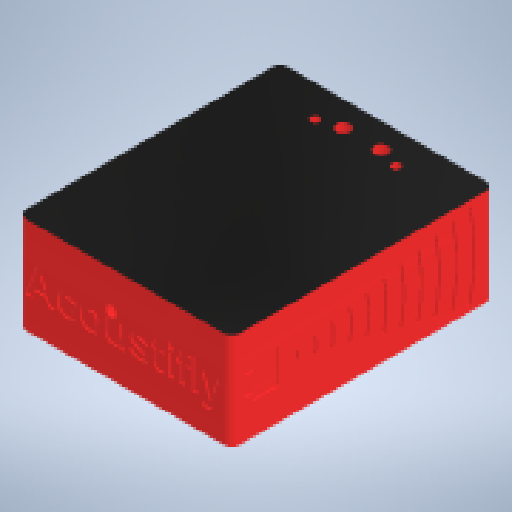
# Autodesk Inventor part: Base
Saved by Autodesk Inventor 2023.3 (Build 273359000, 359)
## iProperties
Created: 2024-05-30
Part Number: Base
Material: Generic
Document SubType Name: Modeling
Designer: Sven
Density: 1 g/cm^3
Appearance: Light Red
Author: Sven
Autodesk Inventor part; units mm, degrees
ref_plane "YZ Plane" through (0, 0, 0) normal (1, 0, 0) x (0, 1, 0)
ref_plane "XZ Plane" through (0, 0, 0) normal (0, 1, 0) x (-1, 0, 0)
ref_plane "XY Plane" through (0, 0, 0) normal (0, 0, 1) x (1, 0, 0)
sketch "Sketch1" plane through (0, 0, 0) normal (0, 1, 0) x (-1, 0, 0)
  line L0 (-25.5, 31.25) -> (25.5, 31.25)
  line L1 (25.5, 31.25) -> (25.5, -31.25)
  line L2 (25.5, -31.25) -> (-25.5, -31.25)
  line L3 (-25.5, -31.25) -> (-25.5, 31.25)
  point P0 (0, 0)
  point P1 (-25.5, 0)
  point P2 (0, -31.25)
  dimension "d0" = 62.5
  dimension "d1" = 51
  constraints: 8 end point, 2 midpoint, 2 parallel, 1 horizontal, 1 horizontal alignment, 1 perpendicular, 1 vertical alignment
  measures "d0" distance of L2.end L0.start
  measures "d1" distance of L1.end L2.end
extrude "Extrusion1" add sketch "Sketch1" along normal blind 23
fillet "Fillet1" radius 2 4 edges at (25.5, 11.5, -31.25) (25.5, 11.5, 31.25) (-25.5, 11.5, -31.25) (-25.5, 11.5, 31.25)
shell "Shell1" thickness 1.8 removed faces 1 at (-8.5, 0, -9.75)
sketch "Sketch2" plane through (-23.5, 21.2, -29.45) normal (0, -1, 0) x (1, 0, 0)
  circle A0 centre (43, 3.2) radius 2
  circle A1 centre (43, 52.2) radius 2
  circle A2 centre (4, 52.2) radius 2
  circle A3 centre (4, 3.2) radius 2
  line L0 (47, -1.8) -> (0, -1.8) projected
  line L1 (0, 60.7) -> (47, 60.7) projected
  line L2 (43, 52.2) -> (4, 52.2)
  line L3 (4, 52.2) -> (4, 3.2)
  line L4 (4, 3.2) -> (43, 3.2)
  line L5 (43, 3.2) -> (43, 52.2)
  line L6 (47, 0) -> (0, 0) projected
  line L7 (0, 58.9) -> (47, 58.9) projected
  line L8 (39, 58.9) -> (39, 52.2)
  line L9 (43, 48.2) -> (47.2, 48.2)
  line L10 (47.2, 58.7) -> (47.2, 0.2) projected
  arc A4 (39, 52.2) -> (43, 48.2) centre (43, 52.2) ccw
  line L11 (8, 58.9) -> (8, 52.2)
  line L12 (-0.2, 48.2) -> (4, 48.2)
  arc A5 (4, 48.2) -> (8, 52.2) centre (4, 52.2) ccw
  line L13 (-0.2, 0.2) -> (-0.2, 58.7) projected
  line L14 (-0.2, 7.2) -> (4, 7.2)
  line L15 (8, 3.2) -> (8, 0)
  arc A6 (8, 3.2) -> (4, 7.2) centre (4, 3.2) ccw
  line L16 (47.2, 7.2) -> (43, 7.2)
  line L17 (39, 0) -> (39, 3.2)
  arc A7 (43, 7.2) -> (39, 3.2) centre (43, 3.2) ccw
  arc A8 (47.2, 58.7) -> (47, 58.9) centre (47, 58.7) ccw projected
  line L18 (47.2, 58.7) -> (47.2, 0.2) projected
  arc A9 (47, 0) -> (47.2, 0.2) centre (47, 0.2) ccw projected
  line L19 (47, 0) -> (0, 0) projected
  arc A10 (-0.2, 0.2) -> (0, 0) centre (0, 0.2) ccw projected
  line L20 (-0.2, 0.2) -> (-0.2, 58.7) projected
  arc A11 (0, 58.9) -> (-0.2, 58.7) centre (0, 58.7) ccw projected
  line L21 (0, 58.9) -> (47, 58.9) projected
  arc A12 (0, 60.7) -> (-2, 58.7) centre (0, 58.7) ccw projected
  line L22 (-2, 0.2) -> (-2, 58.7) projected
  arc A13 (-2, 0.2) -> (0, -1.8) centre (0, 0.2) ccw projected
  line L23 (47, -1.8) -> (0, -1.8) projected
  arc A14 (47, -1.8) -> (49, 0.2) centre (47, 0.2) ccw projected
  line L24 (49, 58.7) -> (49, 0.2) projected
  arc A15 (49, 58.7) -> (47, 60.7) centre (47, 58.7) ccw projected
  line L25 (0, 60.7) -> (47, 60.7) projected
  point P0 (23.5, 29.45)
  point P1 (23.5, 3.2)
  point P2 (23.5, 0)
  point P3 (-0.2, 0.2)
  point P4 (47.2, 0.2)
  point P5 (47, 58.9)
  point P6 (0, 58.9)
  point P7 (-0.2, 58.7)
  dimension "d6" = 4
  dimension "d7" = 5
  dimension "d9" = 8.5
  dimension "d10" = 39
  dimension "d11" = 2
  dimension "d12" = 2
  dimension "d13" = 2
  dimension "d14" = 2
  constraints: 24 end point, 15 point on line, 8 centre point, 8 perpendicular, 8 point on circle, 4 concentric, 3 equal radius, 2 coincident, 2 horizontal, 2 horizontal alignment, 2 midpoint, 2 parallel, 2 vertical alignment
  measures "d6" diameter of A1
  measures "d7" distance from line of L0 A0.centre
  measures "d9" distance from line of L1 L2.start
  measures "d10" distance of L2.start L2.end
  measures "d11" radial gap between concentric circles of A4 A1
  measures "d12" radial gap between concentric circles of A2 A5
  measures "d13" radial gap between concentric circles of A3 A6
  measures "d14" radial gap between concentric circles of A7 A0
extrude "Extrusion2" add sketch "Sketch2" along normal blind 4.5 contours A0 L5 L16 L10 A9 L6 L17 L4 | A0 L4 A7 L5 | A4 L2 A1 L5 | L5 A1 L2 L8 L7 A8 L10 L9 | L15 L6 A10 L13 L14 L3 A3 L4 | L4 A3 L3 A6 | A5 L3 A2 L2 | L2 A2 L3 L12 L13 A11 L7 L11
sketch "Sketch3" plane through (23.5, 0, -31.25) normal (0, 0, -1) x (-1, 0, 0)
  line L0 (17.3204, 15.3186) -> (10.8612, 15.3213)
  arc A0 (10.8612, 15.3213) -> (9.405, 13.995) centre (10.8606, 13.8594) ccw
  line L1 (9.405, 13.995) -> (9.405, 13.0849)
  arc A1 (9.405, 13.0849) -> (10.8624, 11.7368) centre (10.8624, 13.1987) ccw
  line L2 (10.8624, 11.7368) -> (17.4454, 11.7368)
  arc A2 (17.4454, 11.7368) -> (18.7701, 13.0614) centre (17.3031, 13.2038) ccw
  line L3 (18.7701, 13.0614) -> (18.7701, 13.9715)
  arc A3 (18.7701, 13.9715) -> (17.3204, 15.3186) centre (17.3198, 13.8644) ccw
  line L4 (10.8613, 15.7213) -> (17.3206, 15.7186)
  arc A4 (19.1701, 13.9853) -> (17.3206, 15.7186) centre (17.3198, 13.8644) ccw
  line L5 (19.1701, 13.9853) -> (19.1701, 13.0432)
  arc A5 (17.4636, 11.3368) -> (19.1701, 13.0432) centre (17.3031, 13.2038) ccw
  line L6 (17.4636, 11.3368) -> (10.8624, 11.3368)
  arc A6 (9.005, 13.0703) -> (10.8624, 11.3368) centre (10.8624, 13.1987) ccw
  line L7 (9.005, 13.0703) -> (9.005, 14.0124)
  arc A7 (10.8613, 15.7213) -> (9.005, 14.0124) centre (10.8606, 13.8594) ccw
  point P0 (23.5, 0)
  dimension "d20" = 1.4542
  dimension "d21" = 1.4739
  dimension "d22" = 1.4619
  dimension "d23" = 90.024
  dimension "d24" = 9.3651
  dimension "d25" = 4.7299
  dimension "d26" = 11.7368
  dimension "d27" = 15.3161
  dimension "d28" = 2.2346
  dimension "d29" = 1.3246
  dimension "d30" = 1.3246
  dimension "d31" = 7.9077
  dimension "d32" = 7.9089
  dimension "d121" = 0.4
  constraints: 16 end point, 16 point on circle, 8 centre point, 3 tangent, 2 parallel, 2 perpendicular, 1 equal radius, 1 horizontal, 7 other
  measures "d20" radius of A3
  measures "d21" radius of A2
  measures "d22" radius of A1
  measures "d23" angle of L3 L0
  measures "d24" distance between parallel lines of L3 L1
  measures "d25" distance from line of point (23.5, 0) L3
  measures "d26" distance from line of point (23.5, 0) L2
  measures "d27" distance from line of point (23.5, 0) L0
  measures "d28" distance from line of L3.end L2
  measures "d29" distance from line of L3.start L2
  measures "d30" distance from line of L2.end L3
  measures "d31" distance from line of A1.centre L3
  measures "d32" distance from line of L0.end L3
  measures "d121" distance between parallel lines of L0 L4
extrude "Extrusion4" cut sketch "Sketch3" against normal blind 10 contours A3 L3 A2 L2 A1 L1 A0 L0
sketch "Sketch4" plane through (0, 23, 0) normal (0, 1, 0) x (1, 0, 0)
  circle A0 centre (-4.5, 25.25) radius 1.65
  circle A1 centre (4.5, 25.25) radius 1.65
  line L0 (23.5, 31.25) -> (-23.5, 31.25) projected
  line L1 (-4.5, 25.25) -> (4.5, 25.25)
  point P0 (0, 0)
  point P1 (0, 25.25)
  point P2 (0, 31.25)
  dimension "d35" = 3.3
  dimension "d36" = 9
  dimension "d37" = 6
  constraints: 2 centre point, 2 end point, 2 midpoint, 1 equal radius, 1 horizontal, 1 horizontal alignment, 1 vertical alignment
  measures "d35" diameter of A0
  measures "d36" distance of L1.end L1.start
  measures "d37" distance from line of L0 L1.start
extrude "Extrusion5" cut sketch "Sketch4" against normal blind 10
sketch "Sketch5" plane through (23.5, 0, -31.25) normal (0, 0, -1) x (-1, 0, 0)
  line L0 (28.4701, 14.4) -> (35.4701, 14.4)
  line L1 (35.4701, 14.4) -> (35.4701, 10.6)
  line L2 (35.4701, 10.6) -> (28.4701, 10.6)
  line L3 (28.4701, 10.6) -> (28.4701, 14.4)
  line L4 (0, 16.7) -> (8, 16.7) projected
  line L5 (39, 16.7) -> (47, 16.7) projected
  line L6 (18.7701, 13.9715) -> (18.7701, 13.0614) projected
  point P0 (23.5, 0)
  point P1 (18.7701, 13.5164)
  dimension "d40" = 2.3
  dimension "d41" = 6.1
  dimension "d42" = 7
  dimension "d43" = 9.7
  constraints: 8 end point, 2 parallel, 1 horizontal, 1 midpoint, 1 perpendicular
  measures "d40" distance between parallel lines of L5 L0
  measures "d41" distance between parallel lines of L2 L5
  measures "d42" distance of L1.end L2.end
  measures "d43" distance from line of point (18.77, 13.516) L3
extrude "Extrusion6" cut sketch "Sketch5" against normal blind 10
sketch "Sketch6" plane through (23.5, 0, -31.25) normal (0, 0, -1) x (-1, 0, 0)
  circle A0 centre (22.3701, 14.3165) radius 0.75
  line L0 (10.8612, 15.3213) -> (17.3204, 15.3186) projected
  line L1 (18.7701, 13.9715) -> (18.7701, 13.0614) projected
  point P0 (23.5, 0)
  point P1 (18.7701, 13.5164)
  dimension "d46" = 1.5
  dimension "d47" = 1
  dimension "d48" = 3.6
  constraints: 1 centre point, 1 midpoint
  measures "d46" diameter of A0
  measures "d47" distance from line of A0.centre L0
  measures "d48" horizontal distance of point (18.77, 13.516) A0.centre
extrude "Extrusion7" cut sketch "Sketch6" against normal blind 10
sketch "Sketch7" plane through (-23.5, 0, 31.25) normal (0, 0, 1) x (1, 0, 0)
  circle A0 centre (20.2, 14.07) radius 1.25
  line L0 (1, 15.12) -> (7.002, 15.12) projected
  line L1 (0, 16.7) -> (-0.2, 16.7) projected
  line L2 (8, 16.7) -> (0, 16.7) projected
  line L3 (8, 16.7) -> (4, 16.7) projected
  line L4 (4, 16.7) -> (-0.2, 16.7) projected
  line L5 (6, 16.7) -> (2, 16.7) projected
  point P0 (23.5, 0)
  dimension "d51" = 19.2
  dimension "d52" = 2.5
  dimension "d53" = 1.05
  constraints: 1 centre point
  measures "d51" horizontal distance of A0.centre L0.start
  measures "d52" diameter of A0
  measures "d53" distance from line of A0.centre L0
extrude "Extrusion8" cut sketch "Sketch7" against normal blind 10
sketch "Sketch8" plane through (0, 0, 0) normal (0, -1, 0) x (1, 0, 0)
  line L0 (23.5, -29.45) -> (-23.5, -29.45) projected
  line L1 (19.2, -29.45) -> (23.7, -24.95)
  line L2 (23.7, 29.25) -> (23.7, -29.25) projected
  arc A0 (23.7, 29.25) -> (23.5, 29.45) centre (23.5, 29.25) ccw projected
  line L3 (23.7, 29.25) -> (23.7, -29.25) projected
  arc A1 (23.5, -29.45) -> (23.7, -29.25) centre (23.5, -29.25) ccw projected
  line L4 (23.5, -29.45) -> (-23.5, -29.45) projected
  arc A2 (-23.7, -29.25) -> (-23.5, -29.45) centre (-23.5, -29.25) ccw projected
  line L5 (-23.7, -29.25) -> (-23.7, 29.25) projected
  arc A3 (-23.5, 29.45) -> (-23.7, 29.25) centre (-23.5, 29.25) ccw projected
  line L6 (-23.5, 29.45) -> (23.5, 29.45) projected
  arc A4 (-23.5, 31.25) -> (-25.5, 29.25) centre (-23.5, 29.25) ccw projected
  line L7 (-25.5, -29.25) -> (-25.5, 29.25) projected
  arc A5 (-25.5, -29.25) -> (-23.5, -31.25) centre (-23.5, -29.25) ccw projected
  line L8 (23.5, -31.25) -> (-23.5, -31.25) projected
  arc A6 (23.5, -31.25) -> (25.5, -29.25) centre (23.5, -29.25) ccw projected
  line L9 (25.5, 29.25) -> (25.5, -29.25) projected
  arc A7 (25.5, 29.25) -> (23.5, 31.25) centre (23.5, 29.25) ccw projected
  line L10 (-23.5, 31.25) -> (23.5, 31.25) projected
  line L11 (23.7, 24.95) -> (19.2, 29.45)
  line L12 (-23.7, 24.95) -> (-19.2, 29.45)
  line L13 (-19.2, -29.45) -> (-23.7, -24.95)
  point P0 (0, 0)
  point P1 (23.7, -29.25)
  point P2 (-19.2, -29.45)
  dimension "d56" = 4.5
  dimension "d57" = 4.5
  dimension "d58" = 4.5
  dimension "d59" = 4.5
  dimension "d60" = 4.5
  dimension "d61" = 4.5
  dimension "d62" = 4.5
  dimension "d63" = 4.5
  constraints: 8 end point, 8 point on line
  measures "d56" distance from line of L2 L1.start
  measures "d57" distance from line of L0 L1.end
  measures "d58" distance from line of L6 L11.start
  measures "d59" distance from line of L2 L11.end
  measures "d60" distance from line of L5 L12.end
  measures "d61" distance from line of L6 L12.start
  measures "d62" distance from line of L5 L13.start
  measures "d63" distance from line of L0 L13.end
extrude "Extrusion9" add sketch "Sketch8" against normal blind 4 contours L0 L1 L2 A1 | L0 A2 L5 L13 | L11 L6 A0 L2 | L5 A3 L6 L12
sketch "Sketch9" plane through (0, 0, 0) normal (0, -1, 0) x (1, 0, 0)
  line L0 (-23.7, -29.25) -> (-23.7, -22.25) projected
  arc A0 (-23.7, -29.25) -> (-23.5, -29.45) centre (-23.5, -29.25) ccw projected
  line L1 (-15.5, -29.45) -> (-23.5, -29.45) projected
  line L2 (-15.5, -29.45) -> (-15.5, -26.25) projected
  arc A1 (-15.5, -26.25) -> (-19.5, -22.25) centre (-19.5, -26.25) ccw projected
  line L3 (-19.5, -22.25) -> (-23.7, -22.25) projected
  circle A2 centre (-19.5, -26.25) radius 2 projected
  line L4 (23.7, 24.95) -> (23.7, -24.95) projected
  line L5 (23.7, -24.95) -> (19.2, -29.45) projected
  line L6 (19.2, -29.45) -> (-19.2, -29.45) projected
  line L7 (-19.2, -29.45) -> (-23.7, -24.95) projected
  line L8 (-23.7, -24.95) -> (-23.7, 24.95) projected
  line L9 (-23.7, 24.95) -> (-19.2, 29.45) projected
  line L10 (-19.2, 29.45) -> (19.2, 29.45) projected
  line L11 (19.2, 29.45) -> (23.7, 24.95) projected
  arc A3 (-23.5, 31.25) -> (-25.5, 29.25) centre (-23.5, 29.25) ccw projected
  line L12 (-25.5, -29.25) -> (-25.5, 29.25) projected
  arc A4 (-25.5, -29.25) -> (-23.5, -31.25) centre (-23.5, -29.25) ccw projected
  line L13 (23.5, -31.25) -> (-23.5, -31.25) projected
  arc A5 (23.5, -31.25) -> (25.5, -29.25) centre (23.5, -29.25) ccw projected
  line L14 (25.5, 29.25) -> (25.5, -29.25) projected
  arc A6 (25.5, 29.25) -> (23.5, 31.25) centre (23.5, 29.25) ccw projected
  line L15 (-23.5, 31.25) -> (23.5, 31.25) projected
  line L16 (23.5, -29.45) -> (15.5, -29.45) projected
  arc A7 (23.5, -29.45) -> (23.7, -29.25) centre (23.5, -29.25) ccw projected
  line L17 (23.7, -22.25) -> (23.7, -29.25) projected
  line L18 (23.7, -22.25) -> (19.5, -22.25) projected
  arc A8 (19.5, -22.25) -> (15.5, -26.25) centre (19.5, -26.25) ccw projected
  line L19 (15.5, -26.25) -> (15.5, -29.45) projected
  circle A9 centre (19.5, -26.25) radius 2 projected
  line L20 (23.7, 29.25) -> (23.7, 18.75) projected
  arc A10 (23.7, 29.25) -> (23.5, 29.45) centre (23.5, 29.25) ccw projected
  line L21 (15.5, 29.45) -> (23.5, 29.45) projected
  line L22 (15.5, 29.45) -> (15.5, 22.75) projected
  arc A11 (15.5, 22.75) -> (19.5, 18.75) centre (19.5, 22.75) ccw projected
  line L23 (19.5, 18.75) -> (23.7, 18.75) projected
  circle A12 centre (19.5, 22.75) radius 2 projected
  line L24 (-23.5, 29.45) -> (-15.5, 29.45) projected
  arc A13 (-23.5, 29.45) -> (-23.7, 29.25) centre (-23.5, 29.25) ccw projected
  line L25 (-23.7, 18.75) -> (-23.7, 29.25) projected
  line L26 (-23.7, 18.75) -> (-19.5, 18.75) projected
  arc A14 (-19.5, 18.75) -> (-15.5, 22.75) centre (-19.5, 22.75) ccw projected
  line L27 (-15.5, 22.75) -> (-15.5, 29.45) projected
  circle A15 centre (-19.5, 22.75) radius 2 projected
  point P0 (0, 0)
  point P1 (23.7, -24.95)
  point P2 (19.2, -29.45)
  point P3 (19.2, 29.45)
  point P4 (-19.2, 29.45)
extrude "Extrusion10" cut sketch "Sketch9" against normal blind 2 contours L0 L7 L1 A0 | L25 A13 L24 L9 | L5 L17 A7 L16 | L21 A10 L20 L11
sketch "Sketch12" plane through (0, 23, 0) normal (0, 1, 0) x (1, 0, 0)
  circle A0 centre (-9.6, 23.75) radius 1.1 projected
  circle A1 centre (9.6, 23.75) radius 1.1 projected
  point P0 (0, 0)
extrude "Extrusion13" cut sketch "Sketch12" against normal through all
sketch "Sketch10" plane through (-23.5, 0, 31.25) normal (0, 0, 1) x (1, 0, 0)
  line L0 (-0.133, 14.659) -> (47.133, 14.659) construction
  line L1 (47.133, 14.659) -> (47.133, 5.4822) construction
  line L2 (47.133, 5.4822) -> (-0.133, 5.4822) construction
  line L3 (-0.133, 5.4822) -> (-0.133, 14.659) construction
  line L4 (0, 23) -> (47, 23) projected
  line L5 (6.8883, 7.5417) -> (5.3518, 7.5417)
  line L6 (5.3518, 7.5417) -> (4.7435, 9.1316)
  line L7 (4.7435, 9.1316) -> (1.9478, 9.1316)
  line L8 (1.9478, 9.1316) -> (1.3662, 7.5417)
  line L9 (1.3662, 7.5417) -> (-0.133, 7.5417)
  line L10 (-0.133, 7.5417) -> (2.588, 14.5417)
  line L11 (2.588, 14.5417) -> (4.0926, 14.5417)
  line L12 (4.0926, 14.5417) -> (6.8883, 7.5417)
  line L13 (4.29, 10.3161) -> (3.3243, 12.909)
  line L14 (3.3243, 12.909) -> (2.3746, 10.3161)
  line L15 (2.3746, 10.3161) -> (4.29, 10.3161)
  line L16 (12.0476, 11.1164) -> (10.7245, 10.8763)
  spline S0 degree 2 poles (10.7245, 10.8763) (10.6604, 11.2711) (10.1856, 11.6712) (9.8068, 11.6712) knots 0 0 0 1 2 2 2
  spline S1 degree 2 poles (9.8068, 11.6712) (9.3106, 11.6712) (8.713, 10.9776) (8.713, 10.1667) knots 0 0 0 1 2 2 2
  spline S2 degree 2 poles (8.713, 10.1667) (8.713, 9.265) (9.3213, 8.5234) (9.8281, 8.5234) knots 0 0 0 1 2 2 2
  spline S3 degree 2 poles (9.8281, 8.5234) (10.2123, 8.5234) (10.6978, 8.9609) (10.7992, 9.4891) knots 0 0 0 1 2 2 2
  line L17 (10.7992, 9.4891) -> (12.117, 9.265)
  spline S4 degree 2 poles (12.117, 9.265) (11.9143, 8.358) (10.7458, 7.4296) (9.7694, 7.4296) knots 0 0 0 1 2 2 2
  spline S5 degree 2 poles (9.7694, 7.4296) (8.6597, 7.4296) (7.3365, 8.8328) (7.3365, 10.076) knots 0 0 0 1 2 2 2
  spline S6 degree 2 poles (7.3365, 10.076) (7.3365, 11.3298) (8.6597, 12.7276) (9.7908, 12.7276) knots 0 0 0 1 2 2 2
  spline S7 degree 2 poles (9.7908, 12.7276) (10.7191, 12.7276) (11.8075, 11.9327) (12.0476, 11.1164) knots 0 0 0 1 2 2 2
  spline S8 degree 2 poles (12.7572, 10.1507) (12.7572, 10.8176) (13.4188, 12.0714) (14.6246, 12.7276) (15.3716, 12.7276) knots 0 0 0 1 2 3 3 3
  spline S9 degree 2 poles (15.3716, 12.7276) (16.524, 12.7276) (17.9966, 11.2337) (17.9966, 10.092) knots 0 0 0 1 2 2 2
  spline S10 degree 2 poles (17.9966, 10.092) (17.9966, 8.9449) (16.508, 7.4296) (15.3822, 7.4296) knots 0 0 0 1 2 2 2
  spline S11 degree 2 poles (15.3822, 7.4296) (14.6833, 7.4296) (13.4188, 8.0592) (12.7572, 9.2757) (12.7572, 10.1507) knots 0 0 0 1 2 3 3 3
  spline S12 degree 2 poles (14.1338, 10.0813) (14.1338, 9.3237) (14.8487, 8.5234) (15.3769, 8.5234) knots 0 0 0 1 2 2 2
  spline S13 degree 2 poles (15.3769, 8.5234) (15.9051, 8.5234) (16.6147, 9.3237) (16.6147, 10.0866) knots 0 0 0 1 2 2 2
  spline S14 degree 2 poles (16.6147, 10.0866) (16.6147, 10.8336) (15.9051, 11.6339) (15.3769, 11.6339) knots 0 0 0 1 2 2 2
  spline S15 degree 2 poles (15.3769, 11.6339) (14.8487, 11.6339) (14.1338, 10.8336) (14.1338, 10.0813) knots 0 0 0 1 2 2 2
  line L18 (22.3822, 7.5417) -> (22.3822, 8.2993)
  spline S16 degree 2 poles (22.3822, 8.2993) (22.1048, 7.8938) (21.2031, 7.4296) (20.7016, 7.4296) knots 0 0 0 1 2 2 2
  spline S17 degree 2 poles (20.7016, 7.4296) (20.1894, 7.4296) (19.3784, 7.8778) (19.0156, 8.6888) (19.0156, 9.409) knots 0 0 0 1 2 3 3 3
  line L19 (19.0156, 9.409) -> (19.0156, 12.6156)
  line L20 (19.0156, 12.6156) -> (20.3601, 12.6156)
  line L21 (20.3601, 12.6156) -> (20.3601, 10.284)
  spline S18 degree 2 poles (20.3601, 10.284) (20.3601, 9.217) (20.5095, 8.7368) (20.899, 8.454) (21.1978, 8.454) knots 0 0 0 1 2 3 3 3
  spline S19 degree 2 poles (21.1978, 8.454) (21.5446, 8.454) (22.0835, 8.8328) (22.2862, 9.3877) (22.2862, 10.4761) knots 0 0 0 1 2 3 3 3
  line L22 (22.2862, 10.4761) -> (22.2862, 12.6156)
  line L23 (22.2862, 12.6156) -> (23.6307, 12.6156)
  line L24 (23.6307, 12.6156) -> (23.6307, 7.5417)
  line L25 (23.6307, 7.5417) -> (22.3822, 7.5417)
  line L26 (24.5484, 8.9929) -> (25.8929, 9.1956)
  spline S20 degree 2 poles (25.8929, 9.1956) (25.9783, 8.8061) (26.5065, 8.4007) (26.976, 8.4007) knots 0 0 0 1 2 2 2
  spline S21 degree 2 poles (26.976, 8.4007) (27.4989, 8.4007) (27.7603, 8.5927) knots 0 0 0 1 1 1
  spline S22 degree 2 poles (27.7603, 8.5927) (27.9364, 8.7261) (27.9364, 8.9502) knots 0 0 0 1 1 1
  spline S23 degree 2 poles (27.9364, 8.9502) (27.9364, 9.0996) (27.8403, 9.201) knots 0 0 0 1 1 1
  spline S24 degree 2 poles (27.8403, 9.201) (27.7389, 9.297) (27.3921, 9.377) knots 0 0 0 1 1 1
  spline S25 degree 2 poles (27.3921, 9.377) (25.7702, 9.7345) (25.338, 10.0333) knots 0 0 0 1 1 1
  spline S26 degree 2 poles (25.338, 10.0333) (24.7351, 10.4441) (24.7351, 11.1697) knots 0 0 0 1 1 1
  spline S27 degree 2 poles (24.7351, 11.1697) (24.7351, 11.8313) (25.7755, 12.7276) (26.8693, 12.7276) knots 0 0 0 1 2 2 2
  spline S28 degree 2 poles (26.8693, 12.7276) (27.9097, 12.7276) (28.9181, 12.05) (29.1101, 11.3831) knots 0 0 0 1 2 2 2
  line L27 (29.1101, 11.3831) -> (27.8457, 11.1484)
  spline S29 degree 2 poles (27.8457, 11.1484) (27.7656, 11.4472) (27.3121, 11.7619) (26.8906, 11.7619) knots 0 0 0 1 2 2 2
  spline S30 degree 2 poles (26.8906, 11.7619) (26.3624, 11.7619) (26.1383, 11.6125) knots 0 0 0 1 1 1
  spline S31 degree 2 poles (26.1383, 11.6125) (25.9836, 11.5112) (25.9836, 11.3404) knots 0 0 0 1 1 1
  spline S32 degree 2 poles (25.9836, 11.3404) (25.9836, 11.2017) (26.117, 11.1004) knots 0 0 0 1 1 1
  spline S33 degree 2 poles (26.117, 11.1004) (26.2984, 10.967) (28.4379, 10.4815) (28.8594, 10.124) knots 0 0 0 1 2 2 2
  spline S34 degree 2 poles (28.8594, 10.124) (29.2809, 9.7665) (29.2809, 9.1263) knots 0 0 0 1 1 1
  spline S35 degree 2 poles (29.2809, 9.1263) (29.2809, 8.4327) (28.1178, 7.4296) (26.976, 7.4296) knots 0 0 0 1 2 2 2
  spline S36 degree 2 poles (26.976, 7.4296) (25.9409, 7.4296) (24.7351, 8.2726) (24.5484, 8.9929) knots 0 0 0 1 2 2 2
  line L28 (32.7809, 12.6156) -> (32.7809, 11.5485)
  line L29 (32.7809, 11.5485) -> (31.8632, 11.5485)
  line L30 (31.8632, 11.5485) -> (31.8632, 9.5051)
  spline S37 degree 2 poles (31.8632, 9.5051) (31.8632, 8.8862) (31.9165, 8.6781) (32.1033, 8.5447) (32.2367, 8.5447) knots 0 0 0 1 2 3 3 3
  spline S38 degree 2 poles (32.2367, 8.5447) (32.4234, 8.5447) (32.7809, 8.6728) knots 0 0 0 1 1 1
  line L31 (32.7809, 8.6728) -> (32.8929, 7.6324)
  spline S39 degree 2 poles (32.8929, 7.6324) (32.4234, 7.4296) (31.8312, 7.4296) knots 0 0 0 1 1 1
  spline S40 degree 2 poles (31.8312, 7.4296) (31.4684, 7.4296) (30.8868, 7.675) (30.6147, 8.0592) (30.5614, 8.39) knots 0 0 0 1 2 3 3 3
  spline S41 degree 2 poles (30.5614, 8.39) (30.5187, 8.6247) (30.5187, 9.3343) knots 0 0 0 1 1 1
  line L32 (30.5187, 9.3343) -> (30.5187, 11.5485)
  line L33 (30.5187, 11.5485) -> (29.9051, 11.5485)
  line L34 (29.9051, 11.5485) -> (29.9051, 12.6156)
  line L35 (29.9051, 12.6156) -> (30.5187, 12.6156)
  line L36 (30.5187, 12.6156) -> (30.5187, 13.624)
  line L37 (30.5187, 13.624) -> (31.8632, 14.4136)
  line L38 (31.8632, 14.4136) -> (31.8632, 12.6156)
  line L39 (31.8632, 12.6156) -> (32.7809, 12.6156)
  line L40 (33.7146, 7.5417) -> (33.7146, 12.6156)
  line L41 (33.7146, 12.6156) -> (35.0591, 12.6156)
  line L42 (35.0591, 12.6156) -> (35.0591, 7.5417)
  line L43 (35.0591, 7.5417) -> (33.7146, 7.5417)
  line L44 (33.7146, 13.2985) -> (33.7146, 14.5417)
  line L45 (33.7146, 14.5417) -> (35.0591, 14.5417)
  line L46 (35.0591, 14.5417) -> (35.0591, 13.2985)
  line L47 (35.0591, 13.2985) -> (33.7146, 13.2985)
  line L48 (35.838, 12.6156) -> (36.585, 12.6156)
  line L49 (36.585, 12.6156) -> (36.585, 12.9944)
  spline S42 degree 2 poles (36.585, 12.9944) (36.585, 13.6347) (36.8571, 14.2642) (37.588, 14.659) (38.1482, 14.659) knots 0 0 0 1 2 3 3 3
  spline S43 degree 2 poles (38.1482, 14.659) (38.7245, 14.659) (39.274, 14.4883) knots 0 0 0 1 1 1
  line L50 (39.274, 14.4883) -> (39.0926, 13.56)
  spline S44 degree 2 poles (39.0926, 13.56) (38.7725, 13.6347) (38.4737, 13.6347) knots 0 0 0 1 1 1
  spline S45 degree 2 poles (38.4737, 13.6347) (38.1803, 13.6347) (37.9295, 13.3625) (37.9295, 12.9731) knots 0 0 0 1 2 2 2
  line L51 (37.9295, 12.9731) -> (37.9295, 12.6156)
  line L52 (37.9295, 12.6156) -> (38.9325, 12.6156)
  line L53 (38.9325, 12.6156) -> (38.9325, 11.5592)
  line L54 (38.9325, 11.5592) -> (37.9295, 11.5592)
  line L55 (37.9295, 11.5592) -> (37.9295, 7.5417)
  line L56 (37.9295, 7.5417) -> (36.585, 7.5417)
  line L57 (36.585, 7.5417) -> (36.585, 11.5592)
  line L58 (36.585, 11.5592) -> (35.838, 11.5592)
  line L59 (35.838, 11.5592) -> (35.838, 12.6156)
  line L60 (39.6848, 7.5417) -> (39.6848, 14.5417)
  line L61 (39.6848, 14.5417) -> (41.0293, 14.5417)
  line L62 (41.0293, 14.5417) -> (41.0293, 7.5417)
  line L63 (41.0293, 7.5417) -> (39.6848, 7.5417)
  line L64 (41.7656, 12.6156) -> (43.1955, 12.6156)
  line L65 (43.1955, 12.6156) -> (44.412, 9.0142)
  line L66 (44.412, 9.0142) -> (45.5911, 12.6156)
  line L67 (45.5911, 12.6156) -> (46.9783, 12.6156)
  line L68 (46.9783, 12.6156) -> (45.1963, 7.7284)
  line L69 (45.1963, 7.7284) -> (44.8708, 6.8481)
  spline S46 degree 2 poles (44.8708, 6.8481) (44.6947, 6.4052) (44.3746, 5.9357) (43.9585, 5.6423) (43.3502, 5.4822) (42.9661, 5.4822) knots 0 0 0 1 2 3 4 4 4
  spline S47 degree 2 poles (42.9661, 5.4822) (42.5819, 5.4822) (42.2085, 5.5622) knots 0 0 0 1 1 1
  line L70 (42.2085, 5.5622) -> (42.0911, 6.6133)
  spline S48 degree 2 poles (42.0911, 6.6133) (42.4059, 6.5493) (42.662, 6.5493) knots 0 0 0 1 1 1
  spline S49 degree 2 poles (42.662, 6.5493) (43.1261, 6.5493) (43.5796, 7.0988) (43.697, 7.5257) knots 0 0 0 1 2 2 2
  line L71 (43.697, 7.5257) -> (41.7656, 12.6156)
  point P0 (23.5, 0)
  point P1 (23.5, 14.659)
  point P2 (23.5, 23)
  dimension "d0" = 62.5
  dimension "d1" = 51
  dimension "d68" = 47.266
  dimension "d69" = 9.1768
  dimension "d70" = 8.341
  constraints: 2 midpoint, 1 vertical alignment, 2 other
  measures "d68" distance of L1.end L2.end
  measures "d69" distance of L2.end L0.start
  measures "d70" distance between parallel lines of L4 L0
extrude "Extrusion11" cut sketch "Sketch10" against normal blind 0.4
sketch "Sketch11" plane through (25.5, 0, 29.25) normal (1, 0, 0) x (0, 0, -1)
  line L0 (9.25, 7.75) -> (9.25, 15.25)
  line L1 (9, 15.5) -> (3.25, 15.5)
  line L2 (3, 15.25) -> (3, 7.75)
  line L3 (3.25, 7.5) -> (9, 7.5)
  arc A0 (3.25, 15.5) -> (3, 15.25) centre (3.25, 15.25) ccw
  arc A1 (9.25, 15.25) -> (9, 15.5) centre (9, 15.25) ccw
  arc A2 (9, 7.5) -> (9.25, 7.75) centre (9, 7.75) ccw
  arc A3 (3, 7.75) -> (3.25, 7.5) centre (3.25, 7.75) ccw
  line L4 (3, 14) -> (1, 14)
  line L5 (1, 14) -> (1, 13.5)
  line L6 (1, 13.5) -> (3, 13.5)
  line L7 (3, 9.5) -> (1, 9.5)
  line L8 (1, 9.5) -> (1, 9)
  line L9 (1, 9) -> (3, 9)
  circle A4 centre (9.25, 11.5) radius 4.2
  circle A5 centre (9.25, 11.5) radius 4.7
  circle A6 centre (9.25, 11.5) radius 8.4
  circle A7 centre (9.25, 11.5) radius 8.9
  circle A8 centre (9.25, 11.5) radius 12.6
  circle A9 centre (9.25, 11.5) radius 13.1
  circle A10 centre (9.25, 11.5) radius 16.8
  circle A11 centre (9.25, 11.5) radius 17.3
  circle A12 centre (9.25, 11.5) radius 21
  circle A13 centre (9.25, 11.5) radius 21.5
  circle A14 centre (9.25, 11.5) radius 25.2
  circle A15 centre (9.25, 11.5) radius 25.7
  circle A16 centre (9.25, 11.5) radius 29.4
  circle A17 centre (9.25, 11.5) radius 29.9
  circle A18 centre (9.25, 11.5) radius 33.6
  circle A19 centre (9.25, 11.5) radius 34.1
  circle A20 centre (9.25, 11.5) radius 37.8
  circle A21 centre (9.25, 11.5) radius 38.3
  circle A22 centre (9.25, 11.5) radius 42
  circle A23 centre (9.25, 11.5) radius 42.5
  circle A24 centre (9.25, 11.5) radius 46.2
  circle A25 centre (9.25, 11.5) radius 46.7
  line L10 (0, 0) -> (58.5, 0) projected
  line L11 (0, 23) -> (58.5, 23) projected
  line L12 (60.5, 0) -> (60.5, 23) projected
  line L13 (9.25, 11.5) -> (60.5, 23)
  line L14 (9.25, 11.5) -> (60.5, 0)
  point P0 (29.25, 0)
  point P1 (-7, 28.5)
  point P2 (9.25, 7.5)
  point P3 (3, 15.5)
  point P4 (9.25, 15.5)
  point P5 (9.25, 11.5)
  point P6 (1, 13.75)
  point P7 (13.3481, 10.5804)
  point P8 (13.836, 10.471)
  point P9 (13.836, 12.529)
  point P10 (13.3481, 12.4196)
  point P11 (17.4462, 9.6609)
  point P12 (17.9341, 9.5514)
  point P13 (17.9341, 13.4486)
  point P14 (17.4462, 13.3391)
  point P15 (21.5443, 8.7413)
  point P16 (22.0322, 8.6318)
  point P17 (22.0322, 14.3682)
  point P18 (21.5443, 14.2587)
  point P19 (25.6424, 7.8217)
  point P20 (26.1303, 7.7122)
  point P21 (26.1303, 15.2878)
  point P22 (25.6424, 15.1783)
  point P23 (29.7405, 6.9021)
  point P24 (30.2283, 6.7927)
  point P25 (30.2283, 16.2073)
  point P26 (29.7405, 16.0979)
  point P27 (33.8386, 5.9826)
  point P28 (34.3264, 5.8731)
  point P29 (34.3264, 17.1269)
  point P30 (33.8386, 17.0174)
  point P31 (37.9367, 5.063)
  point P32 (38.4245, 4.9535)
  point P33 (38.4245, 18.0465)
  point P34 (37.9367, 17.937)
  point P35 (42.0348, 4.1434)
  point P36 (42.5226, 4.0339)
  point P37 (42.5226, 18.9661)
  point P38 (42.0348, 18.8566)
  point P39 (46.1329, 3.2238)
  point P40 (46.6207, 3.1144)
  point P41 (46.6207, 19.8856)
  point P42 (46.1329, 19.7762)
  point P43 (50.231, 2.3043)
  point P44 (50.7188, 2.1948)
  point P45 (50.7188, 20.8052)
  point P46 (50.231, 20.6957)
  point P47 (54.329, 1.3847)
  point P48 (54.8169, 1.2752)
  point P49 (54.8169, 21.7248)
  point P50 (54.329, 21.6153)
  dimension "d73" = 6.25
  dimension "d74" = 8
  dimension "d78" = 0.25
  dimension "d79" = 0.5
  dimension "d80" = 0.5
  dimension "d81" = 2
  dimension "d82" = 1.5
  dimension "d83" = 1.5
  dimension "d84" = 8.4
  dimension "d85" = 9.4
  dimension "d86" = 16.8
  dimension "d87" = 17.8
  dimension "d88" = 25.2
  dimension "d89" = 26.2
  dimension "d90" = 33.6
  dimension "d91" = 34.6
  dimension "d92" = 42
  dimension "d93" = 43
  dimension "d94" = 50.4
  dimension "d95" = 51.4
  dimension "d96" = 58.8
  dimension "d97" = 59.8
  dimension "d98" = 67.2
  dimension "d99" = 68.2
  dimension "d100" = 75.6
  dimension "d101" = 76.6
  dimension "d102" = 84
  dimension "d103" = 85
  dimension "d104" = 92.4
  dimension "d105" = 93.4
  dimension "d108" = 23
  dimension "d109" = 11.5
  dimension "d110" = 1
  dimension "d111" = 67.5
  dimension "d112" = 5.5
  constraints: 26 centre point, 22 coincident, 20 end point, 12 point on line, 8 point on circle, 8 tangent, 4 parallel, 4 perpendicular, 3 equal radius, 2 midpoint, 6 other
  measures "d73" distance of point (9.25, 15.5) point (3, 15.5)
  measures "d74" distance of point (9.25, 7.5) point (9.25, 15.5)
  measures "d78" radius of A0
  measures "d79" distance of L7.end L9.start
  measures "d80" distance of L4.end L5.end
  measures "d81" distance of L5.end L6.end
  measures "d82" distance between parallel lines of L9 L3
  measures "d83" distance between parallel lines of L4 L1
  measures "d84" diameter of A4
  measures "d85" diameter of A5
  measures "d86" diameter of A6
  measures "d87" diameter of A7
  measures "d88" diameter of A8
  measures "d89" diameter of A9
  measures "d90" diameter of A10
  measures "d91" diameter of A11
  measures "d92" diameter of A12
  measures "d93" diameter of A13
  measures "d94" diameter of A14
  measures "d95" diameter of A15
  measures "d96" diameter of A16
  measures "d97" diameter of A17
  measures "d98" diameter of A18
  measures "d99" diameter of A19
  measures "d100" diameter of A20
  measures "d101" diameter of A21
  measures "d102" diameter of A22
  measures "d103" diameter of A23
  measures "d104" diameter of A24
  measures "d105" diameter of A25
  measures "d108" distance between parallel lines of L10 L11
  measures "d109" distance from line of point (9.25, 11.5) L11
  measures "d110" horizontal distance of L11.start point (1, 13.75)
  measures "d111" distance from line of point (-7, 28.5) L12
  measures "d112" distance from line of point (-7, 28.5) L11
extrude "Extrusion12" cut sketch "Sketch11" against normal blind 0.4 contours A2 L3 A4 L1 A1 L0 | L13 A5 L14 A4 | L3 A5 L1 A4 | L3 A3 L2 A0 L1 A5 | L13 A7 L14 A6 | A6 L6 L5 L4 | L4 L2 L6 A6 | A6 L7 L2 L9 | L9 L8 L7 A6 | L13 A9 L14 A8 | L13 A11 L14 A10 | L13 A13 L14 A12 | L13 A15 L14 A14 | L13 A17 L14 A16 | L13 A19 L14 A18 | L13 A21 L14 A20 | L13 A23 L14 A22 | L13 A25 L14 A24
mirror "Mirror1" about plane through (0, 0, 0) normal (1, 0, 0) of "Extrusion12"
sketch "Sketch13" plane through (23.5, 0, -31.25) normal (0, 0, -1) x (-1, 0, 0)
  circle A0 centre (23.5, 6) radius 1.6
  circle A1 centre (23.5, 6) radius 2 projected
  point P0 (23.5, 0)
  dimension "d117" = 3.2
  constraints: 1 centre point, 1 concentric
  measures "d117" diameter of A0
extrude "Extrusion14" cut sketch "Sketch13" against normal blind 10 contours A0
sketch "Sketch14" plane through (23.5, 0, -31.25) normal (0, 0, -1) x (-1, 0, 0)
  circle A0 centre (23.5, 6) radius 1.6 projected
  circle A1 centre (22.3701, 14.3165) radius 0.75 projected
  line L0 (35.4701, 14.4) -> (35.4701, 10.6) projected
  line L1 (35.4701, 10.6) -> (28.4701, 10.6) projected
  line L2 (28.4701, 10.6) -> (28.4701, 14.4) projected
  line L3 (28.4701, 14.4) -> (35.4701, 14.4) projected
  line L4 (9.405, 13.0849) -> (9.405, 13.995) projected
  arc A2 (10.8612, 15.3213) -> (9.405, 13.995) centre (10.8606, 13.8594) ccw projected
  line L5 (10.8612, 15.3213) -> (17.3204, 15.3186) projected
  arc A3 (18.7701, 13.9715) -> (17.3204, 15.3186) centre (17.3198, 13.8644) ccw projected
  line L6 (18.7701, 13.9715) -> (18.7701, 13.0614) projected
  arc A4 (17.4454, 11.7368) -> (18.7701, 13.0614) centre (17.3031, 13.2038) ccw projected
  line L7 (17.4454, 11.7368) -> (10.8624, 11.7368) projected
  arc A5 (9.405, 13.0849) -> (10.8624, 11.7368) centre (10.8624, 13.1987) ccw projected
  line L8 (47, 23) -> (47, 0) projected
  line L9 (0, 23) -> (47, 23) projected
  line L10 (0, 0) -> (0, 23) projected
  line L11 (0, 0) -> (47, 0) projected
  line L12 (17.3205, 15.5186) -> (10.8613, 15.5213)
  arc A6 (10.8613, 15.5213) -> (9.205, 14.004) centre (10.8606, 13.8594) ccw
  line L13 (9.205, 14.004) -> (9.205, 13.0774)
  arc A7 (9.205, 13.0774) -> (10.8624, 11.5368) centre (10.8624, 13.1987) ccw
  line L14 (10.8624, 11.5368) -> (17.4548, 11.5368)
  arc A8 (17.4548, 11.5368) -> (18.9701, 13.0521) centre (17.3031, 13.2038) ccw
  line L15 (18.9701, 13.0521) -> (18.9701, 13.9786)
  arc A9 (18.9701, 13.9786) -> (17.3205, 15.5186) centre (17.3198, 13.8644) ccw
  point P0 (23.5, 0)
  dimension "d122" = 0.2
  constraints: 8 end point, 8 point on circle, 4 centre point, 7 other
  measures "d122" distance between parallel lines of L5 L12
extrude "Extrusion15" cut sketch "Sketch14" against normal blind 10 contours A9 L15 A8 L14 A7 L13 A6 L12
equation "\"d11\" = d12"
equation "\"d13\" = d12"
equation "\"d14\" = d13"
equation "\"d57\" = d56"
equation "\"d58\" = d57"
equation "\"d59\" = d58"
equation "\"d60\" = d59"
equation "\"d61\" = d60"
equation "\"d62\" = d57"
equation "\"d63\" = d62"
equation "\"d83\" = d82"
body "Solid1"
